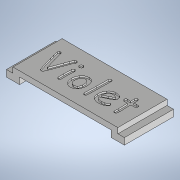
# Autodesk Inventor part: Крышка аккумулятора
Saved by Autodesk Inventor 2020 (Build 240168000, 168)
## iProperties
Created: 2021-04-26
Part Number: Крышка аккумулятора
Material: Типовые
Document SubType Name: Обычные детали
Designer: Антон
Density: 1 g/cm^3
Appearance: По умолчанию
Author: Антон
Autodesk Inventor part; units mm, degrees
ref_plane "YZ Plane" through (0, 0, 0) normal (1, 0, 0) x (0, 1, 0)
ref_plane "XZ Plane" through (0, 0, 0) normal (0, 1, 0) x (-1, 0, 0)
ref_plane "XY Plane" through (0, 0, 0) normal (0, 0, 1) x (1, 0, 0)
sketch "Эскиз1" plane through (0, 0, 0) normal (0, 0, 1) x (1, 0, 0)
  line L0 (0, 0) -> (32, 0)
  line L1 (32, 0) -> (32, 3.65)
  line L2 (32, 3.65) -> (0, 3.65)
  line L3 (0, 3.65) -> (0, 0)
  line L4 (32, 2) -> (34, 2)
  line L5 (34, 2) -> (34, 0)
  line L6 (34, 0) -> (32, 0)
  line L7 (32, 0) -> (32, 2)
  line L8 (-2, 0) -> (0, 0)
  line L9 (0, 0) -> (0, 2)
  line L10 (0, 2) -> (-2, 2)
  line L11 (-2, 2) -> (-2, 0)
  point P0 (0, 2)
  dimension "d32" = 32
  dimension "d33" = 3.65
  dimension "d34" = 2
  dimension "d35" = 2
  constraints: 24 end point, 6 parallel, 4 collinear, 3 horizontal, 3 perpendicular, 2 equal length
  measures "d32" distance of L2.end L1.end
  measures "d33" distance of L1.end L0.end
  measures "d34" distance of L5.end L6.end
  measures "d35" distance of L4.end L5.end
extrude "Выдавливание1" add sketch "Эскиз1" along normal blind 15
sketch "Эскиз9" plane through (0, 0, 15) normal (0, 0, 1) x (1, 0, 0)
  line L0 (0, 3.65) -> (0, 2) projected
  line L1 (32, 3.65) -> (0, 3.65) projected
  line L2 (0, 2) -> (32, 2)
  line L3 (32, 2) -> (32, 3.65)
  line L4 (32, 3.65) -> (0, 3.65)
  line L5 (0, 3.65) -> (0, 2)
  line L6 (-2, 0) -> (34, 0) projected
  line L7 (0, 2) -> (2, 2)
  line L8 (2, 2) -> (2, 0)
  line L9 (2, 0) -> (0, 0)
  line L10 (0, 0) -> (0, 2)
  line L11 (32, 2) -> (32, 3.65) projected
  line L12 (32, 2) -> (30, 2)
  line L13 (30, 2) -> (30, 0)
  line L14 (30, 0) -> (32, 0)
  line L15 (32, 0) -> (32, 2)
  line L16 (34, 2) -> (32, 2) projected
  line L17 (0, 2) -> (-2, 2) projected
  constraints: 24 end point, 6 parallel, 3 horizontal, 3 perpendicular, 2 collinear, 2 point on line
extrude "Выдавливание9" cut sketch "Эскиз9" against normal blind 14 contours L2 L13 L6 L8
sketch "Эскиз8" plane through (0, 3.65, 0) normal (0, 1, 0) x (1, 0, 0)
  line L0 (0, 0) -> (32, 0) construction
  line L1 (32, 0) -> (32, -15) construction
  line L2 (32, -15) -> (0, -15) construction
  line L3 (0, -15) -> (0, 0) construction
  spline S0 degree 2 poles (8.5345, -4.5034) (8.2241, -4.9586) (8.031, -5.4621) knots 0 0 0 1 1 1
  line L4 (8.031, -5.4621) -> (7.6586, -6.5448)
  line L5 (7.6586, -6.5448) -> (6.3276, -10.1448)
  spline S1 degree 2 poles (6.3276, -10.1448) (6.0931, -10.7724) (5.7828, -11.3793) knots 0 0 0 1 1 1
  spline S2 degree 2 poles (5.7828, -11.3793) (5.6241, -11.6759) (5.3345, -11.6759) knots 0 0 0 1 1 1
  spline S3 degree 2 poles (5.3345, -11.6759) (4.9552, -11.6759) (4.8034, -11.2897) knots 0 0 0 1 1 1
  spline S4 degree 2 poles (4.8034, -11.2897) (4.2034, -9.7862) (3.4724, -6.9655) knots 0 0 0 1 1 1
  line L6 (3.4724, -6.9655) -> (3.0793, -5.6)
  spline S5 degree 2 poles (3.0793, -5.6) (2.7897, -4.5724) (2.7897, -4.2552) knots 0 0 0 1 1 1
  spline S6 degree 2 poles (2.7897, -4.2552) (2.7897, -4.0345) (2.9483, -3.8897) knots 0 0 0 1 1 1
  spline S7 degree 2 poles (2.9483, -3.8897) (3.0931, -3.7586) (3.2931, -3.7586) knots 0 0 0 1 1 1
  spline S8 degree 2 poles (3.2931, -3.7586) (3.6724, -3.7586) (3.7759, -4.1655) knots 0 0 0 1 1 1
  line L7 (3.7759, -4.1655) -> (3.9621, -5.0276)
  line L8 (3.9621, -5.0276) -> (4.4379, -6.7034)
  spline S9 degree 2 poles (4.4379, -6.7034) (4.9069, -8.5448) (5.3621, -9.8759) knots 0 0 0 1 1 1
  line L9 (5.3621, -9.8759) -> (5.3897, -9.7931)
  line L10 (5.3897, -9.7931) -> (6.7138, -6.2069)
  line L11 (6.7138, -6.2069) -> (7.1345, -4.9931)
  spline S10 degree 2 poles (7.1345, -4.9931) (7.4172, -4.2621) (7.7345, -3.8897) knots 0 0 0 1 1 1
  spline S11 degree 2 poles (7.7345, -3.8897) (7.9, -3.6897) (8.1207, -3.6897) knots 0 0 0 1 1 1
  spline S12 degree 2 poles (8.1207, -3.6897) (8.3207, -3.6897) (8.631, -3.9931) (8.631, -4.2069) knots 0 0 0 1 2 2 2
  spline S13 degree 2 poles (8.631, -4.2069) (8.631, -4.3517) (8.5345, -4.5034) knots 0 0 0 1 1 1
  spline S14 degree 2 poles (10.5138, -9.0345) (10.5138, -9.331) (10.5483, -10.5172) (10.5483, -10.8138) knots 0 0 0 1 2 2 2
  spline S15 degree 2 poles (10.5483, -10.8138) (10.5483, -11.0345) (10.2793, -11.3103) (10.0655, -11.3103) knots 0 0 0 1 2 2 2
  spline S16 degree 2 poles (10.0655, -11.3103) (9.8517, -11.3103) (9.5759, -11.0345) (9.5759, -10.8138) knots 0 0 0 1 2 2 2
  spline S17 degree 2 poles (9.5759, -10.8138) (9.5759, -10.5172) (9.5414, -9.331) (9.5414, -9.0345) knots 0 0 0 1 2 2 2
  spline S18 degree 2 poles (9.5414, -9.0345) (9.5414, -8.5724) (9.6379, -7.1793) (9.6379, -6.7172) knots 0 0 0 1 2 2 2
  spline S19 degree 2 poles (9.6379, -6.7172) (9.6379, -6.4897) (9.9138, -6.2138) (10.1276, -6.2138) knots 0 0 0 1 2 2 2
  spline S20 degree 2 poles (10.1276, -6.2138) (10.3345, -6.2138) (10.6103, -6.4897) (10.6103, -6.7172) knots 0 0 0 1 2 2 2
  spline S21 degree 2 poles (10.6103, -6.7172) (10.6103, -7.1793) (10.5138, -8.5724) (10.5138, -9.0345) knots 0 0 0 1 2 2 2
  spline S22 degree 2 poles (10.2862, -5.0138) (10.0448, -5.0138) (9.7, -4.6759) (9.7, -4.4414) knots 0 0 0 1 2 2 2
  spline S23 degree 2 poles (9.7, -4.4414) (9.7, -4.2069) (10.0448, -3.869) (10.2862, -3.869) knots 0 0 0 1 2 2 2
  spline S24 degree 2 poles (10.2862, -3.869) (10.5207, -3.869) (10.8655, -4.2069) (10.8655, -4.4414) knots 0 0 0 1 2 2 2
  spline S25 degree 2 poles (10.8655, -4.4414) (10.8655, -4.6759) (10.5207, -5.0138) (10.2862, -5.0138) knots 0 0 0 1 2 2 2
  spline S26 degree 2 poles (14.0517, -11.5724) (13.2241, -11.5724) (12.6241, -10.9586) knots 0 0 0 1 1 1
  spline S27 degree 2 poles (12.6241, -10.9586) (11.9552, -10.2759) (11.9207, -9.1241) knots 0 0 0 1 1 1
  spline S28 degree 2 poles (11.9207, -9.1241) (11.8931, -8.0069) (12.4862, -7.1586) knots 0 0 0 1 1 1
  spline S29 degree 2 poles (12.4862, -7.1586) (13.1759, -6.1517) (14.4103, -6.1517) knots 0 0 0 1 1 1
  spline S30 degree 2 poles (14.4103, -6.1517) (15.4034, -6.1517) (15.9069, -7.0552) knots 0 0 0 1 1 1
  spline S31 degree 2 poles (15.9069, -7.0552) (16.3138, -7.7862) (16.3, -8.8207) knots 0 0 0 1 1 1
  spline S32 degree 2 poles (16.3, -8.8207) (16.2862, -9.9172) (15.7276, -10.6897) knots 0 0 0 1 1 1
  spline S33 degree 2 poles (15.7276, -10.6897) (15.0931, -11.5724) (14.0517, -11.5724) knots 0 0 0 1 1 1
  spline S34 degree 2 poles (14.3483, -7.1586) (13.6241, -7.1517) (13.2172, -7.8483) knots 0 0 0 1 1 1
  spline S35 degree 2 poles (13.2172, -7.8483) (12.8931, -8.4069) (12.8931, -9.1241) knots 0 0 0 1 1 1
  spline S36 degree 2 poles (12.8931, -9.1241) (12.8931, -9.8414) (13.2862, -10.2414) knots 0 0 0 1 1 1
  spline S37 degree 2 poles (13.2862, -10.2414) (13.6103, -10.5724) (14.0517, -10.5724) knots 0 0 0 1 1 1
  spline S38 degree 2 poles (14.0517, -10.5724) (14.569, -10.5724) (14.9345, -10.2) knots 0 0 0 1 1 1
  spline S39 degree 2 poles (14.9345, -10.2) (15.3552, -9.7793) (15.3828, -9.0759) knots 0 0 0 1 1 1
  spline S40 degree 2 poles (15.3828, -9.0759) (15.4517, -7.1655) (14.3483, -7.1586) knots 0 0 0 1 1 1
  line L12 (18.7759, -7.3931) -> (18.7069, -9.8552)
  spline S41 degree 2 poles (18.7069, -9.8552) (18.7069, -10.2483) (18.6655, -11) knots 0 0 0 1 1 1
  spline S42 degree 2 poles (18.6655, -11) (18.6172, -11.4966) (18.1828, -11.4966) knots 0 0 0 1 1 1
  spline S43 degree 2 poles (18.1828, -11.4966) (17.6931, -11.4966) (17.6931, -10.9931) knots 0 0 0 1 1 1
  spline S44 degree 2 poles (17.6931, -10.9931) (17.6931, -10.3931) (17.8034, -7.9931) (17.8034, -7.3931) knots 0 0 0 1 2 2 2
  spline S45 degree 2 poles (17.8034, -7.3931) (17.8034, -6.6138) (17.8517, -4.6) (17.8517, -3.8207) knots 0 0 0 1 2 2 2
  spline S46 degree 2 poles (17.8517, -3.8207) (17.8517, -3.3241) (18.3345, -3.3241) knots 0 0 0 1 1 1
  spline S47 degree 2 poles (18.3345, -3.3241) (18.8241, -3.3241) (18.8241, -3.8207) knots 0 0 0 1 1 1
  spline S48 degree 2 poles (18.8241, -3.8207) (18.8241, -4.6) (18.7759, -6.6138) (18.7759, -7.3931) knots 0 0 0 1 2 2 2
  spline S49 degree 2 poles (22.5966, -11.5103) (21.4793, -11.5103) (20.7897, -10.9517) knots 0 0 0 1 1 1
  spline S50 degree 2 poles (20.7897, -10.9517) (20.031, -10.331) (20.031, -9.2207) knots 0 0 0 1 1 1
  spline S51 degree 2 poles (20.031, -9.2207) (20.031, -7.931) (20.6517, -7.0621) knots 0 0 0 1 1 1
  spline S52 degree 2 poles (20.6517, -7.0621) (21.3345, -6.1103) (22.4655, -6.1103) knots 0 0 0 1 1 1
  spline S53 degree 2 poles (22.4655, -6.1103) (23.2862, -6.1103) (23.8034, -6.3862) knots 0 0 0 1 1 1
  spline S54 degree 2 poles (23.8034, -6.3862) (24.4448, -6.731) (24.4448, -7.4345) knots 0 0 0 1 1 1
  spline S55 degree 2 poles (24.4448, -7.4345) (24.4448, -7.931) (23.8862, -8.3379) knots 0 0 0 1 1 1
  spline S56 degree 2 poles (23.8862, -8.3379) (23.6379, -8.5172) (22.8379, -8.8897) knots 0 0 0 1 1 1
  line L13 (22.8379, -8.8897) -> (20.9483, -9.7862)
  spline S57 degree 2 poles (20.9483, -9.7862) (21.2241, -10.2) (22.0517, -10.6138) (22.5966, -10.6138) knots 0 0 0 1 2 2 2
  spline S58 degree 2 poles (22.5966, -10.6138) (22.9414, -10.6138) (23.3966, -10.4828) knots 0 0 0 1 1 1
  spline S59 degree 2 poles (23.3966, -10.4828) (23.9828, -10.3241) (24.3207, -9.7931) (24.5138, -9.7931) knots 0 0 0 1 2 2 2
  spline S60 degree 2 poles (24.5138, -9.7931) (24.6862, -9.7931) (24.9552, -10.0552) (24.9552, -10.2276) knots 0 0 0 1 2 2 2
  spline S61 degree 2 poles (24.9552, -10.2276) (24.9552, -10.7793) (24.0724, -11.1724) knots 0 0 0 1 1 1
  spline S62 degree 2 poles (24.0724, -11.1724) (23.3138, -11.5103) (22.5966, -11.5103) knots 0 0 0 1 1 1
  spline S63 degree 2 poles (22.4655, -7) (21.8655, -7) (21.0655, -7.9379) (20.8655, -8.8759) knots 0 0 0 1 2 2 2
  line L14 (20.8655, -8.8759) -> (22.3828, -8.1517)
  spline S64 degree 2 poles (22.3828, -8.1517) (23.2793, -7.7172) (23.6586, -7.3931) knots 0 0 0 1 1 1
  spline S65 degree 2 poles (23.6586, -7.3931) (23.231, -7) (22.4655, -7) knots 0 0 0 1 1 1
  spline S66 degree 2 poles (29.1552, -7.069) (29.0517, -7.069) (28.769, -7.0483) (28.6655, -7.0483) knots 0 0 0 1 2 2 2
  spline S67 degree 2 poles (28.6655, -7.0483) (28.5483, -7.0483) (27.9897, -7.1241) knots 0 0 0 1 1 1
  line L15 (27.9897, -7.1241) -> (28.0793, -10.0483)
  line L16 (28.0793, -10.0483) -> (28.0862, -10.2621)
  line L17 (28.0862, -10.2621) -> (28.0931, -10.5172)
  spline S68 degree 2 poles (28.0931, -10.5172) (28.1138, -11.6) (27.5759, -11.6) knots 0 0 0 1 1 1
  spline S69 degree 2 poles (27.5759, -11.6) (27.3759, -11.6) (27.0862, -11.3448) (27.0862, -11.1517) knots 0 0 0 1 2 2 2
  spline S70 degree 2 poles (27.0862, -11.1517) (27.0862, -10.9586) (27.1138, -10.2069) (27.1138, -10.0207) knots 0 0 0 1 2 2 2
  line L18 (27.1138, -10.0207) -> (27.0172, -7.131)
  spline S71 degree 2 poles (27.0172, -7.131) (26.6586, -7.1172) (25.9207, -7.0483) knots 0 0 0 1 1 1
  spline S72 degree 2 poles (25.9207, -7.0483) (25.4793, -6.9862) (25.4793, -6.5586) knots 0 0 0 1 1 1
  spline S73 degree 2 poles (25.4793, -6.5586) (25.4793, -6.3379) (25.7483, -6.0552) (25.9552, -6.0552) knots 0 0 0 1 2 2 2
  line L19 (25.9552, -6.0552) -> (26.9897, -6.1379)
  spline S74 degree 2 poles (26.9897, -6.1379) (26.9897, -5.8828) (26.9483, -5.0414) (26.9483, -4.8552) knots 0 0 0 1 2 2 2
  spline S75 degree 2 poles (26.9483, -4.8552) (26.9483, -4.6414) (27.231, -4.3724) (27.4379, -4.3724) knots 0 0 0 1 2 2 2
  spline S76 degree 2 poles (27.4379, -4.3724) (27.8862, -4.3724) (27.9621, -5.0966) knots 0 0 0 1 1 1
  spline S77 degree 2 poles (27.9621, -5.0966) (27.9759, -5.2828) (27.9759, -5.5379) knots 0 0 0 1 1 1
  line L20 (27.9759, -5.5379) -> (27.969, -5.8276)
  line L21 (27.969, -5.8276) -> (27.9621, -6.131)
  spline S78 degree 2 poles (27.9621, -6.131) (28.5759, -6.0552) (28.6655, -6.0552) knots 0 0 0 1 1 1
  spline S79 degree 2 poles (28.6655, -6.0552) (29.1759, -6.0552) (29.3345, -6.1034) knots 0 0 0 1 1 1
  spline S80 degree 2 poles (29.3345, -6.1034) (29.6379, -6.2) (29.6379, -6.5655) knots 0 0 0 1 1 1
  spline S81 degree 2 poles (29.6379, -6.5655) (29.6379, -6.7862) (29.369, -7.069) (29.1552, -7.069) knots 0 0 0 1 2 2 2
  constraints: 3 coincident, 2 other
emboss "Рельеф1" sketch "Эскиз8" operation cut depth 0.5 direction (0, -1, 0)
equation "\"Радиус_гибки\" = Толщина"
equation "\"Ширина_просечки\" = Толщина"
equation "\"Глубина_просечки\" = 0.5 * Толщина"
equation "\"Размер_просечки\" = 4 * Толщина"
equation "\"Мин_остаток\" = 2 * Толщина"
equation "\"Радиус_перехода\" = Радиус_гибки"
equation "\"Радиус_Якоби\" = Толщина"
equation "\"Размер_зазора\" = Толщина"
equation "\"Толщина\" = 0.5"
